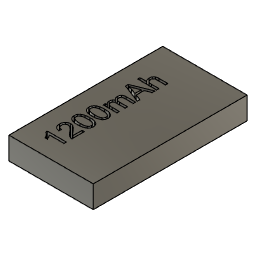
Final HMSU Case Design (Autodesk Fusion 360 archive; units mm, degrees)
design "Battery: 1200mAh"
Autodesk Fusion 360 part; units mm, degrees
sketch "Sketch1" plane through (0, 0, 0) normal (0, 0, 1) x (1, 0, 0)
  line L0 (0, 0) -> (34, 0)
  line L1 (34, 0) -> (34, 62)
  line L2 (34, 62) -> (0, 62)
  line L3 (0, 62) -> (0, 0)
  dimension "d1" = 34
  dimension "d2" = 62
  constraint horizontal L0
  constraint vertical L1
  constraint horizontal L2
  constraint vertical L3
  constraint coincident L0.start L3.end
  measures "d1" distance of L1.end L2.end
  measures "d2" distance of L0.end L1.end
extrude "Extrude1" add sketch "Sketch1" along normal blind 9 makes body 1
sketch "Sketch2" plane through (0, 0, 9) normal (0, 0, 1) x (-1, 0, 0)
  line L0 (0, -62) -> (0, 0)
  line L1 (0, 0) -> (-34, 0)
  line L2 (-34, 0) -> (-34, -62)
  line L3 (-34, -62) -> (0, -62)
  line L4 (-25.4, -6.35) -> (-25.4, -57.15) construction
  line L5 (-25.4, -57.15) -> (-6.35, -57.15) construction
  line L6 (-6.35, -57.15) -> (-6.35, -6.35) construction
  line L7 (-6.35, -6.35) -> (-25.4, -6.35) construction
  text T0 "1200mAh" font "Arial" height 7.62 align left top in box 50.8 x 19.05 at (-25.4, -6.35) x (0, -1) y (1, 0) spacing 1 kerned
extrude "Extrude2" cut sketch "Sketch2" against normal through all text T0 bodies 1 makes body 2 at (9.6767, 18.4375, 4.5) makes body 3 at (9.6767, 24.3578, 4.5) makes body 4 at (10.8409, 40.7838, 6)
